Autodesk Fusion 360 part; units mm, degrees
(part 3 of 3)
equation "d302 = hex_dt_male_depth + slab_dt_fem_depth_tolerance"
equation "d303 = hex_dt_angle"
equation "d304 = hex_dt_male_width_narrower_part + hex_dt_fem_width_tolerance"
equation "d305 = hex_dt_male_depth + slab_dt_fem_depth_tolerance"
equation "d306 = hex_dt_angle"
equation "d307 = slab_base_height"
equation "d310 = hex_top_lip_height"
equation "d4_1 = hex_size_side_to_side"
equation "d16_1 = -hex_top_lip_width"
equation "d29_1 = hex_dt_male_width_narrower_part"
equation "d31_1 = hex_dt_male_depth"
equation "d32_1 = hex_dt_angle"
equation "d34_1 = hex_dt_male_width_narrower_part + hex_dt_fem_width_tolerance"
equation "d35_1 = hex_dt_angle"
equation "d38_1 = hex_multi_store_height"
equation "d44_1 = hex_dt_male_depth + hex_dt_fem_depth_tolerance"
equation "d51_1 = hex_dt_male_bottom_distance + hex_dt_spacing_height_tolerance"
equation "d59_1 = hex_internal_hole_offset"
equation "d313 = -hex_multi_store_male_dt_top_cut_length"
equation "d316 = -hex_top_lip_height"
equation "hex_multi_store_height = ( hex_height * 5 ) - ( hex_top_lip_height * 4 )"
equation "hex_multi_store_male_dt_top_cut_length = ( hex_multi_store_height - hex_height ) + hex_top_lip_height"
equation "d320 = hex_multi_store_internal_hole_height"
equation "hex_multi_store_internal_hole_height = hex_multi_store_height - hex_top_lip_height - 2 mm"
equation "slab_dt_fem_depth_tolerance = 0.2 mm"
equation "d327 = -hex_top_lip_width"
equation "d328 = hex_internal_hole_offset"
equation "d329 = -cap_sculpted_top_wall_thickness"
equation "d330 = hex_size_side_to_side"
equation "d331 = cap_height"
equation "d334 = -cap_top_lip_height"
equation "d327_1 = -hex_top_lip_width"
equation "d328_1 = hex_internal_hole_offset"
equation "d329_1 = -cap_sculpted_top_wall_thickness"
equation "d330_1 = hex_size_side_to_side"
equation "d331_1 = cap_height"
equation "d334_1 = -cap_top_lip_height"
equation "d339_1 = hex_top_lip_height"
equation "cap_road_indent = 0.4 mm" comment "The depth of the pavement part of the road"
equation "d327_2 = -hex_top_lip_width"
equation "d328_2 = hex_internal_hole_offset"
equation "d329_2 = -cap_sculpted_top_wall_thickness"
equation "d330_2 = hex_size_side_to_side"
equation "d331_2 = cap_height"
equation "d334_2 = -cap_top_lip_height"
equation "cap_top_lip_height = 1.8 mm"
equation "d366 = road_total_width"
equation "road_total_width = 10 mm"
equation "road_border_width = 0.4 mm"
equation "d369 = road_border_width"
equation "d370 = -road_border_width"
equation "d372 = -cap_sculpted_hole_depth"
equation "d375 = -cap_road_indent"
equation "d377 = road_total_width"
equation "d378 = road_border_width"
equation "d379 = -road_border_width"
equation "d380 = road_border_width"
equation "d381 = -road_border_width"
equation "road_bridge_pillar_radius = 3 mm"
equation "d383 = road_bridge_pillar_radius"
equation "d384 = road_bridge_pillar_radius"
equation "d385 = cap_top_lip_height"
equation "d387 = cap_top_lip_height"
equation "d390 = -cap_sculpted_hole_depth"
equation "d393 = -cap_road_indent"
equation "d395 = road_total_width / 2"
equation "d396 = -road_total_width / 2"
equation "d397 = -road_border_width"
equation "d398 = road_border_width"
equation "d400 = -cap_sculpted_hole_depth"
equation "d403 = -cap_road_indent"
equation "d327_3 = -hex_top_lip_width"
equation "d328_3 = hex_internal_hole_offset"
equation "d329_3 = -cap_sculpted_top_wall_thickness"
equation "d330_3 = hex_size_side_to_side"
equation "d366_1 = road_total_width"
equation "d369_1 = road_border_width"
equation "d370_1 = -road_border_width"
equation "d405 = road_total_width"
equation "d406 = -road_border_width"
equation "d407 = road_border_width"
equation "d408 = cap_height"
equation "d411 = -cap_top_lip_height"
equation "d414 = -cap_sculpted_hole_depth"
equation "d417 = -cap_road_indent"
equation "d419 = hex_top_lip_height"
equation "d327_3_1 = -hex_top_lip_width"
equation "d328_3_1 = hex_internal_hole_offset"
equation "d329_3_1 = -cap_sculpted_top_wall_thickness"
equation "d330_3_1 = hex_size_side_to_side"
equation "d366_1_1 = road_total_width"
equation "d369_1_1 = road_border_width"
equation "d370_1_1 = -road_border_width"
equation "d408_1 = cap_height"
equation "d411_1 = -cap_top_lip_height"
equation "d419_1 = hex_top_lip_height"
equation "d421 = road_total_width"
equation "d422 = road_border_width"
equation "d423 = -road_border_width"
equation "d425 = -cap_sculpted_hole_depth"
equation "d428 = -cap_road_indent"
equation "d327_3_1_1 = -hex_top_lip_width"
equation "d328_3_1_1 = hex_internal_hole_offset"
equation "d329_3_1_1 = -cap_sculpted_top_wall_thickness"
equation "d330_3_1_1 = hex_size_side_to_side"
equation "d366_1_1_1 = road_total_width"
equation "d369_1_1_1 = road_border_width"
equation "d370_1_1_1 = -road_border_width"
equation "d408_1_1 = cap_height"
equation "d411_1_1 = -cap_top_lip_height"
equation "d419_1_1 = hex_top_lip_height"
equation "d421_1 = road_total_width"
equation "d422_1 = road_border_width"
equation "d423_1 = -road_border_width"
equation "d431 = -cap_sculpted_hole_depth"
equation "d434 = -cap_road_indent"
equation "d327_3_1_1_1 = -hex_top_lip_width"
equation "d328_3_1_1_1 = hex_internal_hole_offset"
equation "d329_3_1_1_1 = -cap_sculpted_top_wall_thickness"
equation "d330_3_1_1_1 = hex_size_side_to_side"
equation "d366_1_1_1_1 = road_total_width"
equation "d369_1_1_1_1 = road_border_width"
equation "d370_1_1_1_1 = -road_border_width"
equation "d408_1_1_1 = cap_height"
equation "d411_1_1_1 = -cap_top_lip_height"
equation "d419_1_1_1 = hex_top_lip_height"
equation "d421_1_1 = road_total_width"
equation "d422_1_1 = road_border_width"
equation "d423_1_1 = -road_border_width"
equation "d436 = road_total_width"
equation "d437 = -road_border_width"
equation "d438 = road_border_width"
equation "d440 = -cap_sculpted_hole_depth"
equation "d443 = -cap_road_indent"
equation "d327_3_1_1_1_1 = -hex_top_lip_width"
equation "d328_3_1_1_1_1 = hex_internal_hole_offset"
equation "d329_3_1_1_1_1 = -cap_sculpted_top_wall_thickness"
equation "d330_3_1_1_1_1 = hex_size_side_to_side"
equation "d366_1_1_1_1_1 = road_total_width"
equation "d369_1_1_1_1_1 = road_border_width"
equation "d370_1_1_1_1_1 = -road_border_width"
equation "d408_1_1_1_1 = cap_height"
equation "d411_1_1_1_1 = -cap_top_lip_height"
equation "d419_1_1_1_1 = hex_top_lip_height"
equation "d421_1_1_1 = road_total_width"
equation "d422_1_1_1 = road_border_width"
equation "d423_1_1_1 = -road_border_width"
equation "d436_1 = road_total_width"
equation "d437_1 = -road_border_width"
equation "d438_1 = road_border_width"
equation "d446 = -cap_sculpted_hole_depth"
equation "d449 = -cap_road_indent"
equation "d327_3_1_1_1_1_1 = -hex_top_lip_width"
equation "d328_3_1_1_1_1_1 = hex_internal_hole_offset"
equation "d329_3_1_1_1_1_1 = -cap_sculpted_top_wall_thickness"
equation "d330_3_1_1_1_1_1 = hex_size_side_to_side"
equation "d366_1_1_1_1_1_1 = road_total_width"
equation "d369_1_1_1_1_1_1 = road_border_width"
equation "d370_1_1_1_1_1_1 = -road_border_width"
equation "d408_1_1_1_1_1 = cap_height"
equation "d411_1_1_1_1_1 = -cap_top_lip_height"
equation "d419_1_1_1_1_1 = hex_top_lip_height"
equation "d421_1_1_1_1 = road_total_width"
equation "d422_1_1_1_1 = road_border_width"
equation "d423_1_1_1_1 = -road_border_width"
equation "d436_1_1 = road_total_width"
equation "d437_1_1 = -road_border_width"
equation "d438_1_1 = road_border_width"
equation "d452 = -cap_sculpted_hole_depth"
equation "d455 = -cap_road_indent"
equation "d327_3_1_1_1_1_1_1 = -hex_top_lip_width"
equation "d328_3_1_1_1_1_1_1 = hex_internal_hole_offset"
equation "d329_3_1_1_1_1_1_1 = -cap_sculpted_top_wall_thickness"
equation "d330_3_1_1_1_1_1_1 = hex_size_side_to_side"
equation "d366_1_1_1_1_1_1_1 = road_total_width"
equation "d369_1_1_1_1_1_1_1 = road_border_width"
equation "d370_1_1_1_1_1_1_1 = -road_border_width"
equation "d408_1_1_1_1_1_1 = cap_height"
equation "d411_1_1_1_1_1_1 = -cap_top_lip_height"
equation "d419_1_1_1_1_1_1 = hex_top_lip_height"
equation "d421_1_1_1_1_1 = road_total_width"
equation "d422_1_1_1_1_1 = road_border_width"
equation "d423_1_1_1_1_1 = -road_border_width"
equation "d436_1_1_1 = road_total_width"
equation "d437_1_1_1 = -road_border_width"
equation "d438_1_1_1 = road_border_width"
equation "d458 = -cap_sculpted_hole_depth"
equation "d461 = -cap_road_indent"
equation "d327_1_1 = -hex_top_lip_width"
equation "d328_1_1 = hex_internal_hole_offset"
equation "d329_1_1 = -cap_sculpted_top_wall_thickness"
equation "d330_1_1 = hex_size_side_to_side"
equation "d464 = road_total_width / 2"
equation "d465 = -road_total_width / 2"
equation "d466 = cap_height"
equation "d469 = -cap_top_lip_height"
equation "d471 = cap_top_lip_height"
equation "d474 = -cap_sculpted_hole_depth"
equation "d476 = road_border_width"
equation "d477 = -road_border_width"
equation "d478 = road_border_width"
equation "d479 = -road_border_width"
equation "d480 = -road_border_width"
equation "d481 = road_border_width"
equation "d483 = -cap_road_indent"
named bodies: "Main Hex Tile", "Basic Cap", "Slab", "Multi Height Hex", "Road Cap", "Road Cap Curve", "Road Cap Bridge", "Road Junction Right", "Road Junction Left", "Road Junction X", "Road Junction Y", "Road Junction Y+I", "Road Junction X + I", "Road Junction 3 Corner", "Curve tight"
